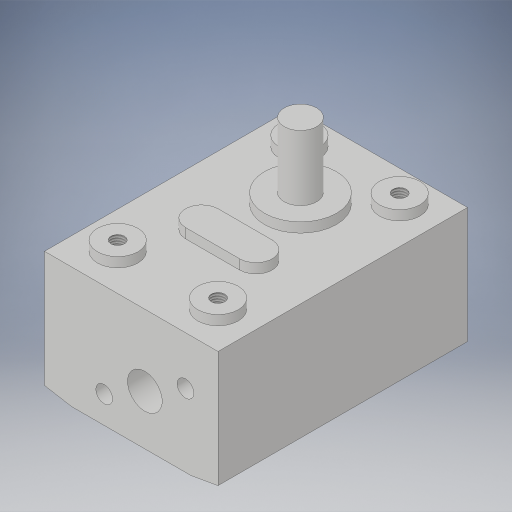
# Autodesk Inventor part: BT803_goteln20_22
Saved by Autodesk Inventor 2023 (Build 270158000, 158)
## iProperties
Company: HTBLA Kaindorf
RuleStatus: InUse
Created: 2023-01-12
Part Number: BT803_goteln20_22
Project: Zeichenmaschine_neu
Material: Generisch
Description: getriebe
Document SubType Name: Modeling
Designer: goteln20
Density: 1 g/cm^3
Appearance: Vorgabe
Mass: 33.0645 g
Surface Area: 74.7289 cm^2
Volume: 33.0645 cm^3
AfterDocNew0: iProperties-Editor_aufrufen
Author: eligo
Keywords: 22
Autodesk Inventor part; units mm, degrees
ref_plane "YZ Plane" through (0, 0, 0) normal (1, 0, 0) x (0, 1, 0)
ref_plane "XZ Plane" through (0, 0, 0) normal (0, 1, 0) x (-1, 0, 0)
ref_plane "XY Plane" through (0, 0, 0) normal (0, 0, 1) x (1, 0, 0)
sketch "Skizze3" plane through (0, 0, 0) normal (0, 0, 1) x (1, 0, 0)
  line L0 (0, 0) -> (-46, 0)
  line L1 (-46, 0) -> (-46, -32)
  line L2 (-46, -32) -> (0, -32)
  line L3 (0, -32) -> (0, 0)
  dimension "d4" = 32
  dimension "d5" = 46
  constraints: 8 end point, 2 parallel, 1 horizontal, 1 perpendicular
  measures "d4" distance of L0.end L1.end
  measures "d5" distance of L1.end L2.end
extrude "Extrusion3" add sketch "Skizze3" along normal blind 22.3
chamfer "Fase1" distance 5 angle 10 2 edges at (-23, -32, 0) (-23, 0, 0) measured on face at (-30.6667, -10.6667, 0)
chamfer "Fase2" distance 5 angle 10 1 edges at (-46, -16, 0) measured on face at (-30.6667, -12.3333, 0)
sketch "Skizze4" plane through (0, -32, 22.3) normal (1, 0, 0) x (0, 0, -1)
  line L0 (21.4184, 32) -> (0, 32) projected
  line L1 (0, 0) -> (0, 32) projected
  line L2 (22.3, 5) -> (22.3, 27) projected
  line L3 (21.4184, 0) -> (0, 0) projected
  point P0 (22.3, 32)
  point P1 (8.9, 26)
  point P2 (17.3, 11)
  point P3 (13.1, 18.5)
  dimension "d17" = 11
  dimension "d18" = 6
  dimension "d19" = 8.9
  dimension "d34" = 9.2
  dimension "d36" = 5
  dimension "d37" = 18.5
  measures "d17" distance from line of L3 point (17.3, 11)
  measures "d18" distance from line of L0 point (8.9, 26)
  measures "d19" distance from line of L1 point (8.9, 26)
  measures "d34" distance from line of point (13.1, 18.5) L2
  measures "d36" distance from line of point (17.3, 11) L2
  measures "d37" distance from line of L3 point (13.1, 18.5)
hole "Bohrung1" at (0, -6, 13.4) at (0, -21, 5) direction (-1, 0, 0) diameter 3.1 depth 8
hole "Bohrung2" at (0, -13.5, 9.2) direction (-1, 0, 0) diameter 6.4 depth 8
sketch "Skizze5" plane through (0, 0, 22.3) normal (0, 0, 1) x (1, 0, 0)
  line L0 (-46, -32) -> (0, -32) projected
  line L1 (0, 0) -> (-46, 0) projected
  line L2 (0, -32) -> (0, 0) projected
  line L3 (-46, 0) -> (-46, -32) projected
  point P0 (-40.25, -25.25)
  point P1 (-40.25, -6.75)
  point P2 (-6.75, -6.75)
  point P3 (-6.75, -25.25)
  point P4 (-31.2, -16)
  point P5 (-46, -16)
  dimension "d38" = 6.75
  dimension "d39" = 6.75
  dimension "d40" = 6.75
  dimension "d41" = 6.75
  dimension "d42" = 6.75
  dimension "d43" = 6.75
  dimension "d44" = 5.75
  dimension "d45" = 5.75
  dimension "d46" = 14.8
  constraints: 1 horizontal alignment, 1 midpoint
  measures "d38" distance from line of L0 point (-40.25, -25.25)
  measures "d39" distance from line of L0 point (-6.75, -25.25)
  measures "d40" distance from line of L1 point (-40.25, -6.75)
  measures "d41" distance from line of L1 point (-6.75, -6.75)
  measures "d42" distance from line of L2 point (-6.75, -6.75)
  measures "d43" distance from line of L2 point (-6.75, -25.25)
  measures "d44" distance from line of L3 point (-40.25, -6.75)
  measures "d45" distance from line of L3 point (-40.25, -25.25)
  measures "d46" distance from line of L3 point (-31.2, -16)
hole "Bohrung3" at (-40.25, -25.25, 22.3) at (-40.25, -6.75, 22.3) at (-6.75, -6.75, 22.3) at (-6.75, -25.25, 22.3) direction (0, 0, -1) diameter 2.5 depth 8
sketch "Skizze6" plane through (0, 0, 22.3) normal (0, 0, 1) x (1, 0, 0)
  circle A0 centre (-40.25, -25.25) radius 1.25 projected
  circle A1 centre (-40.25, -6.75) radius 1.25 projected
  circle A2 centre (-6.75, -6.75) radius 1.25 projected
  circle A3 centre (-6.75, -25.25) radius 1.25 projected
  circle A4 centre (-6.75, -25.25) radius 1.25 projected
  circle A5 centre (-6.75, -25.25) radius 3.75
  circle A6 centre (-6.75, -6.75) radius 3.75
  circle A7 centre (-40.25, -6.75) radius 1.25 projected
  circle A8 centre (-40.25, -6.75) radius 3.75
  circle A9 centre (-40.25, -25.25) radius 3.75
  circle A10 centre (-31.2, -16) radius 6.65
  circle A11 centre (-31.2, -16) radius 3
  line L0 (0, -32) -> (0, 0) projected
  line L1 (-18, -21) -> (-18, -11) construction
  line L2 (-15, -21) -> (-15, -11)
  line L3 (-21, -11) -> (-21, -21)
  arc A12 (-21, -21) -> (-15, -21) centre (-18, -21) ccw
  arc A13 (-15, -11) -> (-21, -11) centre (-18, -11) ccw
  point P0 (-18, -16)
  point P1 (0, -16)
  dimension "d54" = 7.5
  dimension "d55" = 7.5
  dimension "d56" = 7.5
  dimension "d57" = 7.5
  dimension "d58" = 13.3
  dimension "d59" = 6
  dimension "d60" = 18
  dimension "d61" = 10
  dimension "d62" = 6
  constraints: 8 centre point, 8 end point, 6 coincident, 4 point on circle, 4 tangent, 2 midpoint, 1 horizontal alignment, 1 parallel, 1 vertical
  measures "d54" diameter of A9
  measures "d55" diameter of A8
  measures "d56" diameter of A6
  measures "d57" diameter of A5
  measures "d58" diameter of A10
  measures "d59" diameter of A11
  measures "d60" distance from line of L0 point (-18, -16)
  measures "d61" distance of L1.start L1.end
  measures "d62" distance between parallel lines of L3 L2
extrude "Extrusion4" add sketch "Skizze6" along normal blind 1.8 contours A5 | A6 | A8 | A9 | A10 | A11 | A12 L3 A13 L2
thread "Gewinde1" size "M2.5x0.45" class "6H" standard "ISO Metric profile" length 8
thread "Gewinde2" size "M2.5x0.45" class "6H" standard "ISO Metric profile" length 8
thread "Gewinde3" size "M2.5x0.45" class "6H" standard "ISO Metric profile" length 8
thread "Gewinde4" size "M2.5x0.45" class "6H" standard "ISO Metric profile" length 8
extrude "Extrusion5" add sketch "Skizze6" along normal blind 13.8 contours A11
equation "\"d39\" = d38"
equation "\"d40\" = d38"
equation "\"d41\" = d39"
equation "\"d42\" = d41"
equation "\"d43\" = d39"
equation "\"d45\" = d44"
